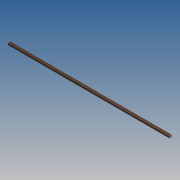
# Autodesk Inventor part: 2h3rbb
Saved by Autodesk Inventor 2014 SP1 (Build 180222100, 222)
## iProperties
Company: HERA Project
Created: 2013-05-20
Part Number: 2h3rbb
Material: Steel, Mild
Document SubType Name: Modeling
Designer: David DeBoer
Density: 7.86 g/cm^3
Description: Hub rebar cross bar
Mass: 236.717 g
Surface Area: 159.005 cm^2
Volume: 30.1167 cm^3
Appearance: Steel
Author: David DeBoer
Title: Hub rebar
Autodesk Inventor part; units mm, degrees
ref_plane "YZ Plane" through (0, 0, 0) normal (1, 0, 0) x (0, 1, 0)
ref_plane "XZ Plane" through (0, 0, 0) normal (0, 1, 0) x (-1, 0, 0)
ref_plane "XY Plane" through (0, 0, 0) normal (0, 0, 1) x (1, 0, 0)
sketch "Sketch2" plane through (0, 0, 0) normal (1, 0, 0) x (0, 1, 0)
  circle A0 centre (0, 0) radius 6
  dimension "d3" = 12
  constraints: 1 centre point, 1 coincident
  measures "d3" diameter of A0
extrude "Extrusion2" add sketch "Sketch2" along normal blind 660.4
body "Solid2"
